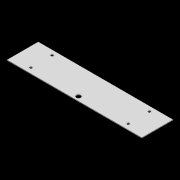
# Autodesk Inventor part: shortsidepanel
Saved by Autodesk Inventor 2022 (Build 260153000, 153)
## iProperties
Created: 2021-10-03
Part Number: shortsidepanel
Material: Generic
Document SubType Name: Modeling
Designer: timmy
Density: 1 g/cm^3
Appearance: Default
Author: timmy
Autodesk Inventor part; units mm, degrees
ref_plane "YZ Plane" through (0, 0, 0) normal (1, 0, 0) x (0, 1, 0)
ref_plane "XZ Plane" through (0, 0, 0) normal (0, 1, 0) x (-1, 0, 0)
ref_plane "XY Plane" through (0, 0, 0) normal (0, 0, 1) x (1, 0, 0)
sketch "Sketch1" plane through (0, 0, 0) normal (0, 1, 0) x (-1, 0, 0)
  line L0 (0, 0) -> (385.572, 0)
  line L1 (385.572, 0) -> (385.572, -89.5604)
  line L2 (385.572, -89.5604) -> (0, -89.5604)
  line L3 (0, -89.5604) -> (0, 0)
  dimension "d0" = 385.572
  dimension "d1" = 89.5604
  constraints: 8 end point, 2 parallel, 1 horizontal, 1 perpendicular
  measures "d0" distance of L1.end L2.end
  measures "d1" distance of L0.end L1.end
extrude "Extrusion1" add sketch "Sketch1" along normal blind 1.5875
sketch "Sketch2" plane through (0, 1.5875, 0) normal (0, 1, 0) x (1, 0, 0)
  line L0 (0, 0) -> (0, 89.5604) projected
  line L1 (-385.572, 0) -> (0, 0) projected
  line L2 (-192.786, 0) -> (-192.786, 32.4011)
  line L3 (-385.572, 89.5604) -> (-385.572, 0) projected
  line L4 (0, 89.5604) -> (-385.572, 89.5604) projected
  line L5 (-331.9526, 89.5604) -> (-318.008, 89.5604) construction
  circle A0 centre (-331.9526, 75.6158) radius 3.175
  circle A1 centre (-331.9526, 14.986) radius 3.175
  circle A2 centre (-53.6194, 75.6158) radius 3.175
  circle A3 centre (-53.6194, 14.986) radius 3.175
  circle A4 centre (-192.786, 11.811) radius 6.35
  constraints: 5 centre point, 4 end point, 2 point on line, 2 symmetric about line, 1 horizontal, 1 midpoint, 1 vertical, 2 other
extrude "Extrusion2" cut sketch "Sketch2" against normal blind 6.35 contours A4 L2 | L2 A4 | A0 | A1 | A2 | A3
equation "\"d7\" = d6"
equation "\"d6\" = 6.35"
body "Solid1"
